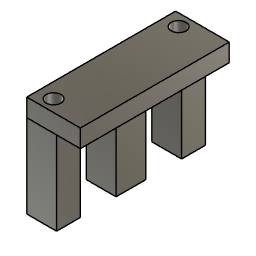
Clip ESP32 v4 (Autodesk Fusion 360 design; units mm, degrees)
Autodesk Fusion 360 part; units mm, degrees
sketch "Sketch1" plane through (0, 0, 0) normal (0, 0, 1) x (1, 0, 0)
  line L0 (0, 0) -> (5, 0)
  line L1 (5, 0) -> (5, 25)
  line L2 (5, 25) -> (0, 25)
  line L3 (0, 25) -> (0, 0)
  circle A0 centre (2.5, 12.5) radius 0.8
  line L4 (0, 10) -> (5, 10)
  line L5 (5, 10) -> (5, 4)
  line L6 (5, 4) -> (0, 4)
  line L7 (0, 4) -> (0, 10)
  line L8 (0, 15) -> (3, 15)
  line L9 (3, 15) -> (3, 14)
  line L10 (3, 14) -> (0, 14)
  line L11 (0, 14) -> (0, 15)
  line L12 (0, 15) -> (5, 15)
  line L13 (5, 15) -> (5, 21)
  line L14 (5, 21) -> (0, 21)
  line L15 (0, 21) -> (0, 15)
  dimension "d1" = 5
  dimension "d2" = 25
  dimension "d3" = 1.6
  dimension "d8" = 6
  dimension "d9" = 6
  constraint horizontal L0
  constraint vertical L1
  constraint horizontal L2
  constraint vertical L3
  constraint coincident L0.start L3.end
  constraint horizontal L4
  constraint vertical L5
  constraint horizontal L6
  constraint vertical L7
  constraint coincident L3 L4.start
  constraint horizontal L8
  constraint vertical L9
  constraint horizontal L10
  constraint vertical L11
  constraint coincident L3 L8.start
  constraint horizontal L12
  constraint vertical L13
  constraint horizontal L14
  constraint vertical L15
  measures "d1" distance of L0.start L0.end
  measures "d2" distance of L0.start L2.end
  measures "d3" diameter of A0
  measures "d8" distance of L4.start L6.end
  measures "d9" distance of L8.start L14.end
extrude "Extrude1" add sketch "Sketch1" along normal blind 14 contours L0 L1 L3 L6 | L1 L3 L4 L5 L6 L7 | L1 L3 L4 L9 L10 L12 | L3 L8 L9 L10 L11 L12 | L1 L3 L8 L12 L13 L14 L15 | L1 L2 L3 L14 | A0 makes body 1
extrude "Extrude2" cut sketch "Sketch1" along normal blind 10 contours A0 bodies 1
extrude "Extrude3" cut sketch "Sketch1" along normal blind 10 contours L1 L3 L8 L12 L13 L14 L15 bodies 1
extrude "Extrude4" cut sketch "Sketch1" along normal blind 10 contours L1 L3 L4 L5 L6 L7 bodies 1
sketch "Sketch2" plane through (0, 0, 14) normal (0, 0, 1) x (-1, 0, 0)
  line L0 (0, -25) -> (0, 0)
  line L1 (0, 0) -> (-5, 0)
  line L2 (-5, 0) -> (-5, -25)
  line L3 (-5, -25) -> (0, -25)
  line L4 (0, -25) -> (-9, -25)
  line L5 (-9, -25) -> (-9, 0)
  line L6 (-9, 0) -> (0, 0)
  line L7 (0, 0) -> (0, -25)
  constraint horizontal L4
  constraint vertical L5
  constraint horizontal L6
  constraint vertical L7
  constraint coincident L0.start L3.end
extrude "Extrude5" add sketch "Sketch2" along normal blind 3 separate body makes body 2
sketch "Sketch3" plane through (0, 0, 17) normal (0, 0, 1) x (-1, 0, 0)
  line L0 (0, 0) -> (-9, 0)
  line L1 (-9, 0) -> (-9, -25)
  line L2 (-9, -25) -> (0, -25)
  line L3 (0, -25) -> (0, 0)
  line L4 (0, 0) -> (-5, 0)
  circle A0 centre (-2.5, -2) radius 0.8
  line L5 (-5, -25) -> (0, -25)
  circle A1 centre (-2.5, -23) radius 0.8
  circle A2 centre (-2.5, -2) radius 1.25
  circle A3 centre (-2.5, -23) radius 1.25
  dimension "d16" = 1.6
  dimension "d18" = 1.6
  dimension "d21" = 2.5
  dimension "d22" = 2.5
  constraint concentric A0 A2
  constraint concentric A1 A3
  measures "d16" diameter of A0
  measures "d18" diameter of A1
  measures "d21" diameter of A2
  measures "d22" diameter of A3
extrude "Extrude6" cut sketch "Sketch3" against normal blind 11 contours A0 | A1 bodies 1 2
extrude "Extrude7" cut sketch "Sketch3" against normal blind 3 contours A1 | A2 bodies 2
extrude "Extrude8" cut sketch "Sketch3" against normal blind 3 contours A3 bodies 2
extrude "Extrude9" add sketch "Sketch3" against normal blind 3 contours A3 bodies 2
extrude "Extrude10" cut sketch "Sketch3" against normal blind 3 contours A3 bodies 2
